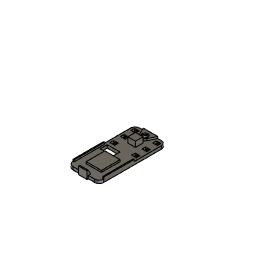
HousingMid (Autodesk Fusion 360 design; units mm, degrees)
Autodesk Fusion 360 part; units mm, degrees
ref_plane "WorkPlane1" through (-4.95, 52.3, -6.5) normal (0, 0, -1) x (-1, 0, 0)
sketch "Sketch1" plane through (8.3, 27.7, -6.5) normal (0, 0, -1) x (1, 0, 0)
  line L0 (-13.25, -24.6) -> (-13.25, 24.6)
  arc A0 (-9.25, 28.6) -> (-13.25, 24.6) centre (-9.25, 24.6) ccw
  line L1 (-9.25, 28.6) -> (-3.475, 28.6)
  line L2 (3.875, 28.6) -> (9.25, 28.6)
  arc A1 (13.25, 24.6) -> (9.25, 28.6) centre (9.25, 24.6) ccw
  line L3 (13.25, 24.6) -> (13.25, -24.6)
  arc A2 (9.25, -28.6) -> (13.25, -24.6) centre (9.25, -24.6) ccw
  line L4 (9.25, -28.6) -> (-9.25, -28.6)
  arc A3 (-13.25, -24.6) -> (-9.25, -28.6) centre (-9.25, -24.6) ccw
  circle A4 centre (0, -23.85) radius 1.5
  line L5 (-3.4, 24.5) -> (-3.4, 30.5) construction
  line L6 (-3.4, 30.5) -> (3.8, 30.5) construction
  line L7 (3.8, 30.5) -> (3.8, 24.5) construction
  line L8 (-3.475, 28.6) -> (-3.4, 28.6)
  line L9 (-3.4, 28.6) -> (-3.4, 29.6)
  line L10 (-3.4, 29.6) -> (3.8, 29.6)
  line L11 (3.8, 29.6) -> (3.8, 28.6)
  line L12 (3.8, 28.6) -> (3.875, 28.6)
  line L13 (-9.75, -23.1) -> (-8.75, -23.1) construction
  line L14 (-8.75, -23.1) -> (-8.75, -26.1) construction
  line L15 (-8.75, -26.1) -> (-9.75, -26.1) construction
  line L16 (-9.75, -26.1) -> (-9.75, -23.1) construction
  line L17 (-9.75, -23.1) -> (-8.75, -26.1) construction
  line L18 (-8.75, -23.1) -> (-9.75, -26.1) construction
  line L19 (-9.75, -23.1) -> (-11.25, -23.1)
  line L20 (-11.25, -23.1) -> (-11.25, -26.1)
  line L21 (-11.25, -26.1) -> (-9.75, -26.1)
  line L22 (-9.75, -26.1) -> (-9.75, -23.1)
  line L23 (-8.75, -23.1) -> (-7.25, -23.1)
  line L24 (-7.25, -23.1) -> (-7.25, -26.1)
  line L25 (-7.25, -26.1) -> (-8.75, -26.1)
  line L26 (-8.75, -26.1) -> (-8.75, -23.1)
  line L27 (-7.25, -17.1) -> (-8.75, -17.1)
  line L28 (-9.75, -17.1) -> (-9.75, -14.1) construction
  line L29 (-9.75, -17.1) -> (-9.75, -14.1)
  line L30 (-8.75, -14.1) -> (-7.25, -14.1)
  line L31 (-8.75, -14.1) -> (-9.75, -17.1) construction
  line L32 (-9.75, -14.1) -> (-11.25, -14.1)
  line L33 (-8.75, -14.1) -> (-8.75, -17.1) construction
  line L34 (-9.75, -14.1) -> (-8.75, -17.1) construction
  line L35 (-8.75, -17.1) -> (-9.75, -17.1) construction
  line L36 (-8.75, -17.1) -> (-8.75, -14.1)
  line L37 (-11.25, -17.1) -> (-9.75, -17.1)
  line L38 (-7.25, -14.1) -> (-7.25, -17.1)
  line L39 (-11.25, -14.1) -> (-11.25, -17.1)
  line L40 (-9.75, -14.1) -> (-8.75, -14.1) construction
  line L41 (-7.25, -8.1) -> (-8.75, -8.1)
  line L42 (-9.75, -8.1) -> (-9.75, -5.1) construction
  line L43 (-9.75, -8.1) -> (-9.75, -5.1)
  line L44 (-8.75, -5.1) -> (-7.25, -5.1)
  line L45 (-8.75, -5.1) -> (-9.75, -8.1) construction
  line L46 (-9.75, -5.1) -> (-11.25, -5.1)
  line L47 (-8.75, -5.1) -> (-8.75, -8.1) construction
  line L48 (-9.75, -5.1) -> (-8.75, -8.1) construction
  line L49 (-8.75, -8.1) -> (-9.75, -8.1) construction
  line L50 (-8.75, -8.1) -> (-8.75, -5.1)
  line L51 (-11.25, -8.1) -> (-9.75, -8.1)
  line L52 (-7.25, -5.1) -> (-7.25, -8.1)
  line L53 (-11.25, -5.1) -> (-11.25, -8.1)
  line L54 (-9.75, -5.1) -> (-8.75, -5.1) construction
  line L55 (0, -15.6) -> (0, -23.85)
  line L56 (11.25, -8.1) -> (9.75, -8.1)
  line L57 (8.75, -8.1) -> (8.75, -5.1)
  line L58 (8.75, -5.1) -> (9.75, -8.1) construction
  line L59 (7.25, -14.1) -> (7.25, -17.1)
  line L60 (8.75, -14.1) -> (8.75, -17.1) construction
  line L61 (11.25, -5.1) -> (11.25, -8.1)
  line L62 (8.75, -8.1) -> (9.75, -8.1) construction
  line L63 (7.25, -17.1) -> (8.75, -17.1)
  line L64 (9.75, -14.1) -> (11.25, -14.1)
  line L65 (9.75, -17.1) -> (9.75, -14.1) construction
  line L66 (7.25, -23.1) -> (7.25, -26.1)
  line L67 (9.75, -5.1) -> (8.75, -8.1) construction
  line L68 (8.75, -23.1) -> (9.75, -26.1) construction
  line L69 (7.25, -8.1) -> (8.75, -8.1)
  line L70 (9.75, -23.1) -> (8.75, -26.1) construction
  line L71 (11.25, -26.1) -> (9.75, -26.1)
  line L72 (8.75, -17.1) -> (9.75, -17.1) construction
  line L73 (9.75, -17.1) -> (9.75, -14.1)
  line L74 (9.75, -8.1) -> (9.75, -5.1)
  line L75 (8.75, -5.1) -> (8.75, -8.1) construction
  line L76 (9.75, -14.1) -> (8.75, -14.1) construction
  line L77 (8.75, -17.1) -> (8.75, -14.1)
  line L78 (7.25, -5.1) -> (7.25, -8.1)
  line L79 (9.75, -5.1) -> (8.75, -5.1) construction
  line L80 (9.75, -8.1) -> (9.75, -5.1) construction
  line L81 (11.25, -17.1) -> (9.75, -17.1)
  line L82 (8.75, -5.1) -> (7.25, -5.1)
  line L83 (8.75, -14.1) -> (9.75, -17.1) construction
  line L84 (9.75, -26.1) -> (9.75, -23.1)
  line L85 (9.75, -23.1) -> (11.25, -23.1)
  line L86 (11.25, -23.1) -> (11.25, -26.1)
  line L87 (9.75, -26.1) -> (9.75, -23.1) construction
  line L88 (11.25, -14.1) -> (11.25, -17.1)
  line L89 (7.25, -26.1) -> (8.75, -26.1)
  line L90 (9.75, -5.1) -> (11.25, -5.1)
  line L91 (8.75, -23.1) -> (8.75, -26.1) construction
  line L92 (8.75, -26.1) -> (9.75, -26.1) construction
  line L93 (9.75, -14.1) -> (8.75, -17.1) construction
  line L94 (8.75, -26.1) -> (8.75, -23.1)
  line L95 (8.75, -23.1) -> (7.25, -23.1)
  line L96 (9.75, -23.1) -> (8.75, -23.1) construction
  line L97 (8.75, -14.1) -> (7.25, -14.1)
  point P0 (-9.25, -24.6)
  point P1 (0, -15.6)
  point P2 (-9.25, -15.6)
  point P3 (-9.25, -15.6)
  point P4 (-9.25, -6.6)
  point P5 (-9.25, -6.6)
  point P6 (9.25, -6.6)
  point P7 (9.25, -24.6)
  point P8 (9.25, -6.6)
  point P9 (9.25, -24.6)
  point P10 (9.25, -15.6)
  point P11 (9.25, -15.6)
  dimension "d50" = 1
  dimension "d51" = 1
  dimension "d52" = 1
  dimension "d53" = 3
  dimension "d54" = 1.5
  dimension "d55" = 3
  dimension "d56" = 1.5
  dimension "d57" = 3
  dimension "d60" = 0
  dimension "d61" = 9
  constraint coincident L1.end L8.start
  constraint coincident L5 L8.end
  constraint perpendicular L5 L8
  constraint perpendicular L8 L9
  constraint coincident L7 L10.end
  constraint perpendicular L7 L10
  constraint perpendicular L10 L11
  constraint coincident L2.start L12.end
  constraint horizontal L13
  constraint perpendicular L13 L14
  constraint parallel L13 L15
  constraint parallel L14 L16
  constraint coincident L17 P0
  constraint coincident L18 P0
  constraint coincident P0 A3.centre
  constraint horizontal L19
  constraint vertical L20
  constraint horizontal L21
  constraint vertical L22
  constraint horizontal L23
  constraint vertical L24
  constraint horizontal L25
  constraint vertical L26
  constraint coincident P1 L55.start
  constraint coincident A4.centre L55.end
  constraint symmetric P0 L55 P9
  constraint symmetric L13.start L55 L70.start
  constraint symmetric L13.end L55 L68.start
  constraint symmetric L14.end L55 L70.end
  constraint symmetric L15.end L55 L68.end
  constraint symmetric L19.end L55 L85.end
  constraint symmetric L20.end L55 L71.start
  constraint symmetric L23.end L55 L66.start
  constraint symmetric L24.end L55 L66.end
  constraint symmetric L27.start L55 L59.end
  constraint symmetric L27.end L55 L60.end
  constraint symmetric L32.end L55 L64.end
  constraint symmetric L28.end L55 L64.start
  constraint symmetric P3 L55 P11
  constraint symmetric L30.end L55 L59.start
  constraint symmetric L28.start L55 L65.start
  constraint symmetric L30.start L55 L60.start
  constraint symmetric L37.start L55 L81.start
  constraint symmetric L41.start L55 L69.start
  constraint symmetric L41.end L55 L57.start
  constraint symmetric L46.end L55 L61.start
  constraint symmetric L42.end L55 L67.start
  constraint symmetric P5 L55 P8
  constraint symmetric L44.end L55 L78.start
  constraint symmetric L42.start L55 L56.end
  constraint symmetric L44.start L55 L57.end
  constraint symmetric L51.start L55 L56.start
  measures "d50" distance of L8.end L9.end
  measures "d51" distance of L10.end L11.end
  measures "d52" distance of L14.end L15.end
  measures "d53" distance of L13.end L14.end
  measures "d54" distance of L13.start L19.end
  measures "d55" distance of L13.start L15.end
  measures "d56" distance of L13.end L23.end
  measures "d57" distance of L13.end L14.end
extrude "Extrude1" add sketch "Sketch1" against normal blind 2
sketch "Sketch2" plane through (0, 0, -4.5) normal (0, 0, 1) x (-1, 0, 0)
  line L0 (2.95, -41.8) -> (2.95, -44.8)
  line L1 (2.95, -44.8) -> (1.45, -44.8)
  line L2 (1.45, -44.8) -> (1.45, -41.8)
  line L3 (1.45, -41.8) -> (2.95, -41.8)
  line L4 (-1.05, -41.8) -> (0.45, -41.8)
  line L5 (0.45, -41.8) -> (0.45, -44.8)
  line L6 (0.45, -44.8) -> (-1.05, -44.8)
  line L7 (-1.05, -44.8) -> (-1.05, -41.8)
  line L8 (0.45, -53.8) -> (-1.05, -53.8)
  line L9 (-1.05, -53.8) -> (-1.05, -50.8)
  line L10 (-1.05, -50.8) -> (0.45, -50.8)
  line L11 (0.45, -50.8) -> (0.45, -53.8)
  line L12 (-1.05, -32.8) -> (0.45, -32.8)
  line L13 (0.45, -32.8) -> (0.45, -35.8)
  line L14 (0.45, -35.8) -> (-1.05, -35.8)
  line L15 (-1.05, -35.8) -> (-1.05, -32.8)
  line L16 (2.95, -32.8) -> (2.95, -35.8)
  line L17 (2.95, -35.8) -> (1.45, -35.8)
  line L18 (1.45, -35.8) -> (1.45, -32.8)
  line L19 (1.45, -32.8) -> (2.95, -32.8)
  line L20 (-17.05, -32.8) -> (-15.55, -32.8)
  line L21 (-15.55, -32.8) -> (-15.55, -35.8)
  line L22 (-15.55, -35.8) -> (-17.05, -35.8)
  line L23 (-17.05, -35.8) -> (-17.05, -32.8)
  circle A0 centre (-8.3, -51.55) radius 1.5
  line L24 (-19.55, -50.8) -> (-18.05, -50.8)
  line L25 (-18.05, -50.8) -> (-18.05, -53.8)
  line L26 (-18.05, -53.8) -> (-19.55, -53.8)
  line L27 (-19.55, -53.8) -> (-19.55, -50.8)
  line L28 (-19.55, -41.8) -> (-18.05, -41.8)
  line L29 (-18.05, -41.8) -> (-18.05, -44.8)
  line L30 (-18.05, -44.8) -> (-19.55, -44.8)
  line L31 (-19.55, -44.8) -> (-19.55, -41.8)
  line L32 (-18.05, -32.8) -> (-18.05, -35.8)
  line L33 (-18.05, -35.8) -> (-19.55, -35.8)
  line L34 (-19.55, -35.8) -> (-19.55, -32.8)
  line L35 (-19.55, -32.8) -> (-18.05, -32.8)
  line L36 (-17.05, -50.8) -> (-15.55, -50.8)
  line L37 (-15.55, -50.8) -> (-15.55, -53.8)
  line L38 (-15.55, -53.8) -> (-17.05, -53.8)
  line L39 (-17.05, -53.8) -> (-17.05, -50.8)
  line L40 (-17.05, -41.8) -> (-15.55, -41.8)
  line L41 (-15.55, -41.8) -> (-15.55, -44.8)
  line L42 (-15.55, -44.8) -> (-17.05, -44.8)
  line L43 (-17.05, -44.8) -> (-17.05, -41.8)
  line L44 (1.45, -53.8) -> (1.45, -50.8)
  line L45 (1.45, -50.8) -> (2.95, -50.8)
  line L46 (2.95, -50.8) -> (2.95, -53.8)
  line L47 (2.95, -53.8) -> (1.45, -53.8)
  arc A1 (4.95, -3.1) -> (0.95, 0.9) centre (0.95, -3.1) ccw
  line L48 (0.95, 0.9) -> (-4.9, 0.9)
  line L49 (-4.9, 0.9) -> (-4.9, 1.9)
  line L50 (-4.9, 1.9) -> (-12.1, 1.9)
  line L51 (-12.1, 1.9) -> (-12.1, 0.9)
  line L52 (-12.1, 0.9) -> (-17.55, 0.9)
  arc A2 (-17.55, 0.9) -> (-21.55, -3.1) centre (-17.55, -3.1) ccw
  line L53 (-21.55, -3.1) -> (-21.55, -52.3)
  arc A3 (-21.55, -52.3) -> (-17.55, -56.3) centre (-17.55, -52.3) ccw
  line L54 (-17.55, -56.3) -> (0.95, -56.3)
  arc A4 (0.95, -56.3) -> (4.95, -52.3) centre (0.95, -52.3) ccw
  line L55 (4.95, -52.3) -> (4.95, -3.1)
  line L56 (1.45, -53.8) -> (0.45, -53.8)
  line L57 (0.45, -50.8) -> (1.45, -50.8)
  line L58 (1.45, -44.8) -> (0.45, -44.8)
  line L59 (0.45, -41.8) -> (1.45, -41.8)
  line L60 (1.45, -35.8) -> (0.45, -35.8)
  line L61 (0.45, -32.8) -> (1.45, -32.8)
  line L62 (-17.05, -35.8) -> (-18.05, -35.8)
  line L63 (-18.05, -32.8) -> (-17.05, -32.8)
  line L64 (-17.05, -41.8) -> (-18.05, -41.8)
  line L65 (-18.05, -44.8) -> (-17.05, -44.8)
  line L66 (-17.05, -53.8) -> (-18.05, -53.8)
  line L67 (-18.05, -50.8) -> (-17.05, -50.8)
  constraint coincident L44.start L47.end
  constraint coincident L8.start L11.end
  constraint coincident L10.end L11.start
  constraint coincident L44.end L45.start
  constraint coincident L1.end L2.start
  constraint coincident L5.end L6.start
  constraint coincident L4.end L5.start
  constraint coincident L2.end L3.start
  constraint coincident L17.end L18.start
  constraint coincident L13.end L14.start
  constraint coincident L12.end L13.start
  constraint coincident L18.end L19.start
  constraint coincident L22.end L23.start
  constraint coincident L32.end L33.start
  constraint coincident L32.start L35.end
  constraint coincident L20.start L23.end
  constraint coincident L40.start L43.end
  constraint coincident L28.end L29.start
  constraint coincident L29.end L30.start
  constraint coincident L42.end L43.start
  constraint coincident L38.end L39.start
  constraint coincident L25.end L26.start
  constraint coincident L24.end L25.start
  constraint coincident L36.start L39.end
extrude "Extrude2" add sketch "Sketch2" along normal blind 0.5
sketch "Sketch3" plane through (0, 0, -4) normal (0, 0, 1) x (-1, 0, 0)
  circle A0 centre (-8.3, -51.55) radius 1.5
  line L0 (-15.55, -44.8) -> (-19.55, -44.8)
  line L1 (-19.55, -44.8) -> (-19.55, -41.8)
  line L2 (-19.55, -41.8) -> (-15.55, -41.8)
  line L3 (-15.55, -41.8) -> (-15.55, -44.8)
  line L4 (-19.55, -32.8) -> (-15.55, -32.8)
  line L5 (-15.55, -32.8) -> (-15.55, -35.8)
  line L6 (-15.55, -35.8) -> (-19.55, -35.8)
  line L7 (-19.55, -35.8) -> (-19.55, -32.8)
  line L8 (-1.05, -41.8) -> (2.95, -41.8)
  line L9 (2.95, -41.8) -> (2.95, -44.8)
  line L10 (2.95, -44.8) -> (-1.05, -44.8)
  line L11 (-1.05, -44.8) -> (-1.05, -41.8)
  line L12 (-1.05, -50.8) -> (2.95, -50.8)
  line L13 (2.95, -50.8) -> (2.95, -53.8)
  line L14 (2.95, -53.8) -> (-1.05, -53.8)
  line L15 (-1.05, -53.8) -> (-1.05, -50.8)
  line L16 (-1.05, -32.8) -> (2.95, -32.8)
  line L17 (2.95, -32.8) -> (2.95, -35.8)
  line L18 (2.95, -35.8) -> (-1.05, -35.8)
  line L19 (-1.05, -35.8) -> (-1.05, -32.8)
  line L20 (-19.55, -50.8) -> (-15.55, -50.8)
  line L21 (-15.55, -50.8) -> (-15.55, -53.8)
  line L22 (-15.55, -53.8) -> (-19.55, -53.8)
  line L23 (-19.55, -53.8) -> (-19.55, -50.8)
  line L24 (4.95, -52.3) -> (4.95, -3.1)
  arc A1 (4.95, -3.1) -> (0.95, 0.9) centre (0.95, -3.1) ccw
  line L25 (0.95, 0.9) -> (-4.9, 0.9)
  line L26 (-4.9, 0.9) -> (-4.9, 1.9)
  line L27 (-4.9, 1.9) -> (-12.1, 1.9)
  line L28 (-12.1, 1.9) -> (-12.1, 0.9)
  line L29 (-12.1, 0.9) -> (-17.55, 0.9)
  arc A2 (-17.55, 0.9) -> (-21.55, -3.1) centre (-17.55, -3.1) ccw
  line L30 (-21.55, -3.1) -> (-21.55, -52.3)
  arc A3 (-21.55, -52.3) -> (-17.55, -56.3) centre (-17.55, -52.3) ccw
  line L31 (-17.55, -56.3) -> (0.95, -56.3)
  arc A4 (0.95, -56.3) -> (4.95, -52.3) centre (0.95, -52.3) ccw
  circle A5 centre (-8.3, -51.55) radius 2.55
  circle A6 centre (-8.3, -51.55) radius 3.55
  circle A7 centre (0.95, -52.3) radius 3
  line L32 (-2.05, -52.3) -> (-2.05, -56.3) construction
  line L33 (-2.05, -56.3) -> (-5.106, -50.0005)
  line L34 (-4.9, 0.9) -> (-12.1, 0.9)
  line L35 (-11.8, -29.2) -> (-19.4, -29.2) construction
  line L36 (-19.4, -29.2) -> (-21.55, -29.2) construction
  line L37 (-21.55, -29.2) -> (-20.55, -29.2)
  line L38 (-21.55, -3.1) -> (-17.55, -3.1) construction
  line L39 (-17.55, -3.1) -> (-17.55, 0.9) construction
  line L40 (-20.55, -29.2) -> (-20.55, -3.1)
  line L41 (-20.55, -3.1) -> (-21.55, -3.1)
  line L42 (-21.55, -3.1) -> (-21.55, -29.2)
  line L43 (-8.3, -51.55) -> (-8.3, -13.31)
  line L44 (-4.8, -29.2) -> (2.8, -29.2) construction
  line L45 (4.95, -29.2) -> (3.95, -29.2)
  arc A8 (4.95, -3.1) -> (0.95, 0.9) centre (0.95, -3.1) ccw
  line L46 (4.95, -3.1) -> (4.95, -29.2)
  line L47 (3.95, -29.2) -> (3.95, -3.1)
  line L48 (4.95, -3.1) -> (0.95, -3.1) construction
  line L49 (4.95, -3.1) -> (4.95, -52.3)
  line L50 (2.8, -29.2) -> (4.95, -29.2) construction
  line L51 (3.95, -3.1) -> (4.95, -3.1)
  line L52 (-14.55, -52.3) -> (-14.55, -56.3) construction
  circle A9 centre (-17.55, -52.3) radius 3
  line L53 (-14.55, -56.3) -> (-11.494, -50.0005)
  point P0 (-15.55, -53.8)
  dimension "d66" = 5.1
  dimension "d67" = 7.1
  dimension "d68" = 1
  constraint concentric A0 A5
  constraint concentric A0 A6
  constraint coincident A7 L32.start
  constraint coincident L31 L32.end
  constraint vertical L32
  constraint tangent A7 L32
  constraint coincident A6 L33.end
  constraint tangent A6 L33
  constraint coincident L25.end L26.start
  constraint coincident L28.end L29.start
  constraint coincident L35.end L36.start
  constraint coincident L30 L36.end
  constraint perpendicular L30 L36
  constraint perpendicular L30 L37
  constraint coincident A2.end L30.start
  constraint coincident A2.centre L38.end
  constraint coincident L29.end A2.start
  constraint coincident L38 L40.end
  constraint perpendicular L38 L40
  constraint coincident A0.centre A5.centre
  constraint vertical L43
  constraint symmetric L14.end L43 P0
  constraint symmetric L29.end L43 A1.end
  constraint symmetric A2.end L43 L24.end
  constraint symmetric A2 L43 A8
  constraint symmetric L30.end L43 L24.start
  constraint symmetric A7 L43 A9
  constraint symmetric L32.start L43 L52.start
  constraint symmetric L32.end L43 L52.end
  constraint symmetric L33.end L43 L53.end
  constraint symmetric L35.start L43 L44.start
  constraint symmetric L35.end L43 L44.end
  constraint symmetric L36.end L43 L45.start
  constraint symmetric L37.end L43 L45.end
  constraint symmetric A2.centre L43 A1.centre
  constraint symmetric L40.end L43 L47.end
  measures "d66" diameter of A5
  measures "d67" diameter of A6
  measures "d68" distance of L36.end L37.end
extrude "Extrude3" add sketch "Sketch3" along normal blind 1.5 contours L24 L45 L46 L47 L49 L51 | L31 A6 L33 L53 | A6 | L26 L27 L28 L34 | L30 L37 L40 L41 L42
extrude "Extrude4" add 1 faces at (7.3, -1.2333, -2.5) along direction (0, 0, 1) blind 2.4
draft "Draft1" angle 30 neutral plane through (0, 0, -0.1) pull (0, 0, 1) 1 faces at (9.7, -0.9, -1.4)
sketch "Sketch4" plane through (0, 0, -4) normal (0, 0, 1) x (-1, 0, 0)
  line L0 (-14.55, -56.3) -> (-11.494, -50.0005)
  arc A0 (-5.106, -50.0005) -> (-11.494, -50.0005) centre (-8.3, -51.55) ccw
  line L1 (-5.106, -50.0005) -> (-2.05, -56.3)
  line L2 (-2.05, -56.3) -> (0.95, -56.3)
  arc A1 (0.95, -56.3) -> (4.95, -52.3) centre (0.95, -52.3) ccw
  line L3 (4.95, -52.3) -> (4.95, -29.2)
  line L4 (4.95, -29.2) -> (3.95, -29.2)
  line L5 (3.95, -29.2) -> (3.95, -3.1)
  line L6 (3.95, -3.1) -> (4.95, -3.1)
  arc A2 (4.95, -3.1) -> (0.95, 0.9) centre (0.95, -3.1) ccw
  line L7 (0.95, 0.9) -> (-4.9, 0.9)
  line L8 (-4.9, 0.9) -> (-4.9, -1.3517)
  line L9 (-4.9, -1.3517) -> (-12.1, -1.3517)
  line L10 (-12.1, -1.3517) -> (-12.1, 0.9)
  line L11 (-12.1, 0.9) -> (-17.55, 0.9)
  arc A3 (-17.55, 0.9) -> (-21.55, -3.1) centre (-17.55, -3.1) ccw
  line L12 (-21.55, -3.1) -> (-20.55, -3.1)
  line L13 (-20.55, -3.1) -> (-20.55, -29.2)
  line L14 (-20.55, -29.2) -> (-21.55, -29.2)
  line L15 (-21.55, -29.2) -> (-21.55, -52.3)
  arc A4 (-21.55, -52.3) -> (-17.55, -56.3) centre (-17.55, -52.3) ccw
  line L16 (-17.55, -56.3) -> (-14.55, -56.3)
  line L17 (-15.55, -44.8) -> (-19.55, -44.8)
  line L18 (-19.55, -44.8) -> (-19.55, -41.8)
  line L19 (-19.55, -41.8) -> (-15.55, -41.8)
  line L20 (-15.55, -41.8) -> (-15.55, -44.8)
  line L21 (-19.55, -32.8) -> (-15.55, -32.8)
  line L22 (-15.55, -32.8) -> (-15.55, -35.8)
  line L23 (-15.55, -35.8) -> (-19.55, -35.8)
  line L24 (-19.55, -35.8) -> (-19.55, -32.8)
  line L25 (-1.05, -41.8) -> (2.95, -41.8)
  line L26 (2.95, -41.8) -> (2.95, -44.8)
  line L27 (2.95, -44.8) -> (-1.05, -44.8)
  line L28 (-1.05, -44.8) -> (-1.05, -41.8)
  line L29 (-1.05, -50.8) -> (2.95, -50.8)
  line L30 (2.95, -50.8) -> (2.95, -53.8)
  line L31 (2.95, -53.8) -> (-1.05, -53.8)
  line L32 (-1.05, -53.8) -> (-1.05, -50.8)
  line L33 (-1.05, -32.8) -> (2.95, -32.8)
  line L34 (2.95, -32.8) -> (2.95, -35.8)
  line L35 (2.95, -35.8) -> (-1.05, -35.8)
  line L36 (-1.05, -35.8) -> (-1.05, -32.8)
  line L37 (-19.55, -50.8) -> (-15.55, -50.8)
  line L38 (-15.55, -50.8) -> (-15.55, -53.8)
  line L39 (-15.55, -53.8) -> (-19.55, -53.8)
  line L40 (-19.55, -53.8) -> (-19.55, -50.8)
  line L41 (-11, -15.5) -> (-11, -8.5) construction
  line L42 (-4, -15.5) -> (-11, -15.5) construction
  line L43 (-11, -8.5) -> (-4, -8.5) construction
  line L44 (-4, -8.5) -> (-4, -15.5) construction
  line L45 (-4, -8.5) -> (-2.5, -8.5) construction
  line L46 (-2.5, -8.5) -> (-2.5, -7) construction
  line L47 (-2.5, -7) -> (-15.5, -7)
  line L48 (-15.5, -7) -> (-15.5, -23)
  line L49 (-15.5, -23) -> (-2.5, -23)
  line L50 (-2.5, -23) -> (-2.5, -7)
  dimension "d75" = 1.5
  dimension "d76" = 1.5
  dimension "d77" = 13
  dimension "d78" = 16
  constraint coincident L43.end L44.start
  constraint perpendicular L44 L45
  constraint perpendicular L45 L46
  constraint horizontal L47
  constraint vertical L48
  constraint horizontal L49
  constraint vertical L50
  measures "d75" distance of L43.end L45.end
  measures "d76" distance of L45.end L46.end
  measures "d77" distance of L46.end L47.end
  measures "d78" distance of L46.end L49.end
extrude "Extrude5" add sketch "Sketch4" along normal blind 1.45 contours L47 L48 L49 L50
sketch "Sketch5" plane through (0, 0, -4) normal (0, 0, 1) x (-1, 0, 0)
  line L0 (-2.5, -23) -> (-15.5, -23)
  line L1 (-15.5, -23) -> (-15.5, -7)
  line L2 (-15.5, -7) -> (-2.5, -7)
  line L3 (-2.5, -7) -> (-2.5, -23)
  line L4 (-14.55, -56.3) -> (-11.494, -50.0005)
  arc A0 (-5.106, -50.0005) -> (-11.494, -50.0005) centre (-8.3, -51.55) ccw
  line L5 (-5.106, -50.0005) -> (-2.05, -56.3)
  line L6 (-2.05, -56.3) -> (0.95, -56.3)
  arc A1 (0.95, -56.3) -> (4.95, -52.3) centre (0.95, -52.3) ccw
  line L7 (4.95, -52.3) -> (4.95, -29.2)
  line L8 (4.95, -29.2) -> (3.95, -29.2)
  line L9 (3.95, -29.2) -> (3.95, -3.1)
  line L10 (3.95, -3.1) -> (4.95, -3.1)
  arc A2 (4.95, -3.1) -> (0.95, 0.9) centre (0.95, -3.1) ccw
  line L11 (0.95, 0.9) -> (-4.9, 0.9)
  line L12 (-4.9, 0.9) -> (-4.9, -1.3517)
  line L13 (-4.9, -1.3517) -> (-12.1, -1.3517)
  line L14 (-12.1, -1.3517) -> (-12.1, 0.9)
  line L15 (-12.1, 0.9) -> (-17.55, 0.9)
  arc A3 (-17.55, 0.9) -> (-21.55, -3.1) centre (-17.55, -3.1) ccw
  line L16 (-21.55, -3.1) -> (-20.55, -3.1)
  line L17 (-20.55, -3.1) -> (-20.55, -29.2)
  line L18 (-20.55, -29.2) -> (-21.55, -29.2)
  line L19 (-21.55, -29.2) -> (-21.55, -52.3)
  arc A4 (-21.55, -52.3) -> (-17.55, -56.3) centre (-17.55, -52.3) ccw
  line L20 (-17.55, -56.3) -> (-14.55, -56.3)
  line L21 (-15.55, -44.8) -> (-19.55, -44.8)
  line L22 (-19.55, -44.8) -> (-19.55, -41.8)
  line L23 (-19.55, -41.8) -> (-15.55, -41.8)
  line L24 (-15.55, -41.8) -> (-15.55, -44.8)
  line L25 (-19.55, -32.8) -> (-15.55, -32.8)
  line L26 (-15.55, -32.8) -> (-15.55, -35.8)
  line L27 (-15.55, -35.8) -> (-19.55, -35.8)
  line L28 (-19.55, -35.8) -> (-19.55, -32.8)
  line L29 (-1.05, -41.8) -> (2.95, -41.8)
  line L30 (2.95, -41.8) -> (2.95, -44.8)
  line L31 (2.95, -44.8) -> (-1.05, -44.8)
  line L32 (-1.05, -44.8) -> (-1.05, -41.8)
  line L33 (-1.05, -50.8) -> (2.95, -50.8)
  line L34 (2.95, -50.8) -> (2.95, -53.8)
  line L35 (2.95, -53.8) -> (-1.05, -53.8)
  line L36 (-1.05, -53.8) -> (-1.05, -50.8)
  line L37 (-1.05, -32.8) -> (2.95, -32.8)
  line L38 (2.95, -32.8) -> (2.95, -35.8)
  line L39 (2.95, -35.8) -> (-1.05, -35.8)
  line L40 (-1.05, -35.8) -> (-1.05, -32.8)
  line L41 (-19.55, -50.8) -> (-15.55, -50.8)
  line L42 (-15.55, -50.8) -> (-15.55, -53.8)
  line L43 (-15.55, -53.8) -> (-19.55, -53.8)
  line L44 (-19.55, -53.8) -> (-19.55, -50.8)
  line L45 (-11.3, -24.65) -> (-11.3, -40.05) construction
  line L46 (-5.3, -40.05) -> (-5.3, -24.65) construction
  line L47 (-17, -28.5) -> (0, -28.5) construction
  line L48 (0, -28.5) -> (0, -5) construction
  line L49 (-17, -5) -> (-17, -28.5) construction
  line L50 (0, -28.5) -> (2.5, -28.5) construction
  line L51 (-5.3, -28.5) -> (-8.3, -28.5) construction
  line L52 (2.5, -28.5) -> (2.5, -24) construction
  line L53 (-8.3, -28.5) -> (-8.3, -30) construction
  line L54 (-8.3, -30) -> (2.5, -30)
  line L55 (2.5, -30) -> (2.5, -24)
  line L56 (2.5, -24) -> (-8.3, -24)
  line L57 (-8.3, -24) -> (-8.3, -30)
  dimension "d81" = 2.5
  dimension "d82" = 3
  dimension "d83" = 4.5
  dimension "d84" = 1.5
  constraint coincident L47.end L48.start
  constraint perpendicular L9 L50
  constraint coincident L46 L51.start
  constraint coincident L47 L51.start
  constraint perpendicular L46 L51
  constraint perpendicular L50 L52
  constraint perpendicular L47 L53
  constraint horizontal L54
  constraint vertical L55
  constraint horizontal L56
  constraint vertical L57
  measures "d81" distance of L47.end L50.end
  measures "d82" distance of L51.start L51.end
  measures "d83" distance of L50.end L52.end
  measures "d84" distance of L51.end L53.end
extrude "Extrude6" cut sketch "Sketch5" against normal through all contours L54 L55 L56 L57
extrude "Extrude8" add 1 faces at (6.1151, 51.3488, -4) along direction (0, 0, 1) blind 0.5
sketch "Sketch7" plane through (0, 0, -4) normal (0, 0, 1) x (-1, 0, 0)
  line L0 (-8.3, -24) -> (2.5, -24)
  line L1 (2.5, -24) -> (2.5, -30)
  line L2 (2.5, -30) -> (-8.3, -30)
  line L3 (-8.3, -30) -> (-8.3, -24)
  line L4 (-2.5, -23) -> (-15.5, -23)
  line L5 (-15.5, -23) -> (-15.5, -7)
  line L6 (-15.5, -7) -> (-2.5, -7)
  line L7 (-2.5, -7) -> (-2.5, -23)
  line L8 (-14.55, -56.3) -> (-11.494, -50.0005)
  arc A0 (-5.106, -50.0005) -> (-11.494, -50.0005) centre (-8.3, -51.55) ccw
  line L9 (-5.106, -50.0005) -> (-2.05, -56.3)
  line L10 (-2.05, -56.3) -> (0.95, -56.3)
  arc A1 (0.95, -56.3) -> (4.95, -52.3) centre (0.95, -52.3) ccw
  line L11 (4.95, -52.3) -> (4.95, -29.2)
  line L12 (4.95, -29.2) -> (3.95, -29.2)
  line L13 (3.95, -29.2) -> (3.95, -3.1)
  line L14 (3.95, -3.1) -> (4.95, -3.1)
  arc A2 (4.95, -3.1) -> (0.95, 0.9) centre (0.95, -3.1) ccw
  line L15 (0.95, 0.9) -> (-4.9, 0.9)
  line L16 (-4.9, 0.9) -> (-4.9, -1.3517)
  line L17 (-4.9, -1.3517) -> (-12.1, -1.3517)
  line L18 (-12.1, -1.3517) -> (-12.1, 0.9)
  line L19 (-12.1, 0.9) -> (-17.55, 0.9)
  arc A3 (-17.55, 0.9) -> (-21.55, -3.1) centre (-17.55, -3.1) ccw
  line L20 (-21.55, -3.1) -> (-20.55, -3.1)
  line L21 (-20.55, -3.1) -> (-20.55, -29.2)
  line L22 (-20.55, -29.2) -> (-21.55, -29.2)
  line L23 (-21.55, -29.2) -> (-21.55, -52.3)
  arc A4 (-21.55, -52.3) -> (-17.55, -56.3) centre (-17.55, -52.3) ccw
  line L24 (-17.55, -56.3) -> (-14.55, -56.3)
  line L25 (-15.55, -44.8) -> (-19.55, -44.8)
  line L26 (-19.55, -44.8) -> (-19.55, -41.8)
  line L27 (-19.55, -41.8) -> (-15.55, -41.8)
  line L28 (-15.55, -41.8) -> (-15.55, -44.8)
  line L29 (-19.55, -32.8) -> (-15.55, -32.8)
  line L30 (-15.55, -32.8) -> (-15.55, -35.8)
  line L31 (-15.55, -35.8) -> (-19.55, -35.8)
  line L32 (-19.55, -35.8) -> (-19.55, -32.8)
  line L33 (-1.05, -41.8) -> (2.95, -41.8)
  line L34 (2.95, -41.8) -> (2.95, -44.8)
  line L35 (2.95, -44.8) -> (-1.05, -44.8)
  line L36 (-1.05, -44.8) -> (-1.05, -41.8)
  line L37 (-1.05, -50.8) -> (2.95, -50.8)
  line L38 (2.95, -50.8) -> (2.95, -53.8)
  line L39 (2.95, -53.8) -> (-1.05, -53.8)
  line L40 (-1.05, -53.8) -> (-1.05, -50.8)
  line L41 (-1.05, -32.8) -> (2.95, -32.8)
  line L42 (2.95, -32.8) -> (2.95, -35.8)
  line L43 (2.95, -35.8) -> (-1.05, -35.8)
  line L44 (-1.05, -35.8) -> (-1.05, -32.8)
  line L45 (-19.55, -50.8) -> (-15.55, -50.8)
  line L46 (-15.55, -50.8) -> (-15.55, -53.8)
  line L47 (-15.55, -53.8) -> (-19.55, -53.8)
  line L48 (-19.55, -53.8) -> (-19.55, -50.8)
  line L49 (-8.3, -46.55) -> (-5.05, -46.55) construction
  line L50 (-5.05, -46.55) -> (-5.05, -43.3) construction
  line L51 (-5.05, -43.3) -> (-5.05, -40.05) construction
  line L52 (-5.05, -40.05) -> (-8.3, -40.05) construction
  line L53 (-8.3, -46.55) -> (-8.3, -40.05) construction
  line L54 (-5.05, -43.3) -> (-8.3, -43.3) construction
  line L55 (-5.05, -46.55) -> (-11.55, -46.55)
  line L56 (-11.55, -46.55) -> (-11.55, -40.05)
  line L57 (-11.55, -40.05) -> (-5.05, -40.05)
  line L58 (-5.05, -40.05) -> (-5.05, -46.55)
  line L59 (-5.05, -46.55) -> (-11.55, -40.05) construction
  line L60 (-11.55, -46.55) -> (-5.05, -40.05) construction
  point P0 (-8.3, -43.3)
  constraint coincident L49.start L53.start
  constraint coincident L52.end L53.end
  constraint coincident L50.end L51.start
  constraint midpoint L53 P0
  constraint horizontal L55
  constraint perpendicular L55 L56
  constraint parallel L55 L57
  constraint parallel L56 L58
  constraint coincident L49.end L50.start
  constraint coincident L59 P0
  constraint coincident L60 P0
  constraint coincident P0 L54.end
extrude "Extrude9" add sketch "Sketch7" along normal blind 4.6 contours L55 L56 L57 L58
move_face "OffsetFaces1" offset -0.1 9 faces at (13.9167, -0.9, -5.6667) (20.6942, 0.6274, -4.8333) (21.55, 28.2, -5.6667) (1, -0.9, -4.8333) (-2.95, -0.3641, -4.8333) (-4.95, 28.2, -5.6667) (-4.8372, 53.243, -4.8333) (10.3833, 56.3, -5.6667) (21.5455, 52.4903, -5.6667)
